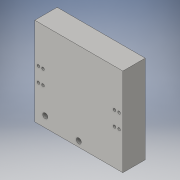
# Autodesk Inventor part: fram jp
Saved by Autodesk Inventor 2016 (Build 200138000, 138)
## iProperties
Created: 2017-09-11
Part Number: fram jp
Material: Generic
Document SubType Name: Modeling
Designer: student
Density: 1 g/cm^3
Appearance: Default
Author: student
Autodesk Inventor part; units mm, degrees
ref_plane "YZ Plane" through (0, 0, 0) normal (1, 0, 0) x (0, 1, 0)
ref_plane "XZ Plane" through (0, 0, 0) normal (0, 1, 0) x (-1, 0, 0)
ref_plane "XY Plane" through (0, 0, 0) normal (0, 0, 1) x (1, 0, 0)
sketch "Sketch1" plane through (0, 0, 0) normal (0, 0, 1) x (1, 0, 0)
  line L0 (-50, -50) -> (50, -50)
  line L1 (50, 50) -> (-50, 50)
  line L2 (-50, 50) -> (-50, -50)
  line L3 (50, -50) -> (-50, 50) construction
  circle A0 centre (0, -43.6681) radius 2.8575
  line L4 (50, 50) -> (50, -50)
  circle A1 centre (-38.091, -38.091) radius 2.8575
  circle A2 centre (40.636, -9.3004) radius 1.5113
  circle A3 centre (45.8176, -9.3004) radius 1.5113
  circle A4 centre (40.636, 7.0318) radius 1.5113
  circle A5 centre (45.8176, 7.0318) radius 1.5113
  circle A6 centre (-45.8176, 7.0318) radius 1.5113
  circle A7 centre (-40.636, 7.0318) radius 1.5113
  circle A8 centre (-45.8176, -9.3004) radius 1.5113
  circle A9 centre (-40.636, -9.3004) radius 1.5113
  dimension "d0" = 100
  dimension "d1" = 100
  dimension "d2" = 5.715
  dimension "d8" = 5.715
  dimension "d19" = 3.0226
  dimension "d24" = 2.159
  dimension "d25" = 13.3096
  constraints: 10 centre point, 10 end point, 1 horizontal, 1 parallel
  measures "d0" distance of L1.start L1.end
  measures "d1" distance of L0.end L1.start
  measures "d2" diameter of A0
  measures "d8" diameter of A1
  measures "d19" diameter of A2
extrude "Extrusion3" add sketch "Sketch1" along normal blind 25.4
body "Solid3"
